Water and power inlet_v8 (Autodesk Fusion 360 design; units mm, degrees)
Autodesk Fusion 360 part; units mm, degrees
sketch "Sketch1" plane through (0, 0, 0) normal (0, 1, 0) x (1, 0, 0)
  line L0 (-30, -30) -> (30, -30)
  line L1 (30, -30) -> (30, 30)
  line L2 (30, 30) -> (-30, 30)
  line L3 (-30, 30) -> (-30, -30)
  line L4 (-30, -30) -> (30, 30) construction
  line L5 (30, -30) -> (-30, 30) construction
  circle A0 centre (10, 0) radius 13.5
  line L6 (10, 0) -> (10, -22.5) construction
  line L7 (10, 0) -> (10, 22.5) construction
  circle A1 centre (10, -22.5) radius 2.25
  circle A2 centre (10, 22.5) radius 2.25
  circle A3 centre (10, 0) radius 17.5
  line L8 (30, -30) -> (24, -30)
  line L9 (24, -30) -> (24, 30)
  line L10 (24, 30) -> (30, 30)
  line L11 (30, 30) -> (30, -30)
  line L12 (-30, -30) -> (-24, -30)
  line L13 (-24, -30) -> (-24, 30)
  line L14 (-24, 30) -> (-30, 30)
  line L15 (-30, 30) -> (-30, -30)
  circle A4 centre (-19, 13) radius 5.6
  line L16 (-11.5, 17.3301) -> (-19, 21.6603)
  line L17 (-19, 21.6603) -> (-26.5, 17.3301)
  line L18 (-26.5, 17.3301) -> (-26.5, 8.6699)
  line L19 (-26.5, 8.6699) -> (-19, 4.3397)
  line L20 (-19, 4.3397) -> (-11.5, 8.6699)
  line L21 (-11.5, 8.6699) -> (-11.5, 17.3301)
  circle A5 centre (10, -22.5) radius 3.75
  circle A6 centre (10, 22.5) radius 3.75
  circle A7 centre (-19, 4.3397) radius 5
  line L22 (-16, 19) -> (-22, 19)
  line L23 (-22, 19) -> (-22, 29)
  line L24 (-22, 29) -> (-16, 29)
  line L25 (-16, 29) -> (-16, 19)
  circle A8 centre (-19, -12) radius 6.25
  line L26 (-28, -27) -> (-10, -27) construction
  line L27 (-10, -27) -> (-10, 3) construction
  line L28 (-10, 3) -> (-28, 3) construction
  line L29 (-28, 3) -> (-28, -27) construction
  line L30 (-28, -27) -> (-10, 3) construction
  line L31 (-10, -27) -> (-28, 3) construction
  circle A9 centre (-10.0486, 22.5) radius 2.55
  circle A10 centre (-10.0486, 22.5) radius 3
  circle A11 centre (-19, -12) radius 10
  line L32 (-22.3912, -17.25) -> (-15.6088, -17.25) construction
  line L33 (-19, -12) -> (-19, -17.25) construction
  line L34 (-19, -17.25) -> (-19.45, -17.25) construction
  line L35 (-19, -17.25) -> (-18.55, -17.25) construction
  line L36 (-18.55, -17.25) -> (-19.45, -17.25)
  line L37 (-19.45, -17.25) -> (-19.45, -18.35)
  line L38 (-19.45, -18.35) -> (-18.55, -18.35)
  line L39 (-18.55, -18.35) -> (-18.55, -17.25)
  point P0 (-19, 13)
  point P1 (-19, -12)
  dimension "d1" = 60
  dimension "d2" = 60
  dimension "d3" = 27
  dimension "d4" = 22.5
  dimension "d5" = 22.5
  dimension "d6" = 4.5
  dimension "d7" = 4.5
  dimension "d18" = 35
  dimension "d19" = 6
  dimension "d20" = 6
  dimension "d24" = 11.2
  dimension "d34" = 7.5
  dimension "d35" = 7.5
  dimension "d36" = 7.5
  dimension "d73" = 10
  dimension "d74" = 12.5
  dimension "d75" = 18
  dimension "d76" = 30
  dimension "d77" = 6
  dimension "d78" = 5.1
  dimension "d85" = 6
  dimension "d91" = 20
  dimension "d92" = 5.25
  dimension "d93" = 0.45
  dimension "d94" = 0.45
  dimension "d95" = 1.1
  constraint horizontal L0
  constraint perpendicular L0 L1
  constraint parallel L0 L2
  constraint parallel L1 L3
  constraint coincident L4 origin
  constraint coincident L5 origin
  constraint coincident A0.centre L6.start
  constraint vertical L6
  constraint parallel L6 L7
  constraint coincident L6.end A1.centre
  constraint coincident L7.end A2.centre
  constraint concentric A0 A3
  constraint horizontal L8
  constraint vertical L9
  constraint horizontal L10
  constraint vertical L11
  constraint horizontal L12
  constraint vertical L13
  constraint horizontal L14
  constraint vertical L15
  constraint coincident P0 A4.centre
  constraint concentric A2 A6
  constraint coincident L19.end L20.start
  constraint tangent L13 A7
  constraint horizontal L22
  constraint vertical L23
  constraint horizontal L24
  constraint vertical L25
  constraint horizontal L26
  constraint perpendicular L26 L27
  constraint parallel L26 L28
  constraint parallel L27 L29
  constraint coincident L30 P1
  constraint coincident L31 P1
  constraint coincident P1 A8.centre
  constraint concentric A9 A10
  constraint concentric A8 A11
  constraint coincident A8 L32.start
  constraint coincident A8 L32.end
  constraint horizontal L32
  constraint midpoint L32 L33.end
  constraint perpendicular L33 L34
  constraint perpendicular L33 L35
  constraint horizontal L36
  constraint vertical L37
  constraint horizontal L38
  constraint vertical L39
  measures "d1" distance of L1.end L2.end
  measures "d2" distance of L0.end L1.end L2.end
  measures "d3" diameter of A0
  measures "d4" distance of A0.centre L6.end
  measures "d5" distance of A0.centre L7.end
  measures "d6" diameter of A1
  measures "d7" diameter of A2
  measures "d18" diameter of A3
  measures "d19" distance of L0.end L8.end
  measures "d20" distance of L0.start L12.end L2.end
  measures "d24" diameter of A4
  measures "d34" distance of P0 L21
  measures "d35" diameter of A5
  measures "d36" diameter of A6
  measures "d73" distance of L22.start L24.end
  measures "d74" diameter of A8
  measures "d75" distance of L27.end L28.end
  measures "d76" distance of L26.end L27.end
  measures "d77" distance of P0 L22
  measures "d78" diameter of A9
  measures "d85" diameter of A10
  measures "d91" diameter of A11
  measures "d92" distance of P1 L32
  measures "d93" distance of L33.end L34.end
  measures "d94" distance of L33.end L35.end
  measures "d95" distance of L35.end L38.end
extrude "Extrude1" add sketch "Sketch1" along normal blind 14 contours L0 L2 L3 L12 L13 L14 L15 L17 L18 L19 A11 | L0 L2 A3 L9 L13 L16 L17 L20 L21 A7 L23 L24 L25 A11 | L0 L1 L2 A3 L8 L9 L10 L11 | L13 A8 A11 | L13 A8 A11 L37 L38 L39 | A3 L9 | A3 L9 | L13 A8 | L13 A8 L36 L37 L39 | A8 L36 L37 L39 | A8 L37 L38 L39 | L13 L19 A7 | A5 | A6 | A9 | A10
sketch "Sketch2" plane through (0, 0, 30) normal (0, 0, 1) x (-1, 0, 0)
  line L0 (-30, 0) -> (-30, -14)
  line L1 (-30, -14) -> (30, -14)
  line L2 (30, -14) -> (30, 0)
  line L3 (31.85, 1.95) -> (33.4186, 1.95)
  line L4 (30.114, 0.8971) -> (31.423, -0.4137)
  arc A0 (31.423, -0.4137) -> (31.85, -0.2372) centre (31.6, -0.2372) ccw
  line L5 (31.85, -8.95) -> (31.85, -6.7628)
  line L6 (33.4186, -8.95) -> (31.85, -8.95)
  line L7 (36.05, -6.3186) -> (33.4186, -8.95)
  line L8 (31.85, -0.2372) -> (31.85, 1.95)
  arc A1 (31.85, -6.7628) -> (31.4232, -6.5861) centre (31.6, -6.7628) ccw
  line L9 (31.4232, -6.5861) -> (30.1424, -7.8668)
  line L10 (33.4186, 1.95) -> (36.05, -0.6814)
  line L11 (36.05, -0.6814) -> (36.05, -6.3186)
  line L12 (30.1571, -7.8522) -> (30, -7.8522)
  line L13 (30, -7.8522) -> (30, 0.8812)
  line L14 (30, 0.8812) -> (30.1299, 0.8812)
  line L15 (40, -9) -> (-35, -9) construction
  line L16 (0, -16) -> (0, 2) construction
  line L17 (-30.114, 0.8971) -> (-31.423, -0.4137)
  line L18 (-31.85, -0.2372) -> (-31.85, 1.95)
  line L19 (-31.4232, -6.5861) -> (-30.1424, -7.8668)
  line L20 (-30, 0.8812) -> (-30.1299, 0.8812)
  line L21 (-30.1571, -7.8522) -> (-30, -7.8522)
  line L22 (-33.4186, 1.95) -> (-36.05, -0.6814)
  line L23 (-31.85, 1.95) -> (-33.4186, 1.95)
  line L24 (-33.4186, -8.95) -> (-31.85, -8.95)
  line L25 (-31.85, -8.95) -> (-31.85, -6.7628)
  arc A2 (-31.85, -0.2372) -> (-31.423, -0.4137) centre (-31.6, -0.2372) ccw
  line L26 (-30, -7.8522) -> (-30, 0.8812)
  line L27 (-36.05, -6.3186) -> (-33.4186, -8.95)
  line L28 (-36.05, -0.6814) -> (-36.05, -6.3186)
  arc A3 (-31.4232, -6.5861) -> (-31.85, -6.7628) centre (-31.6, -6.7628) ccw
  point P0 (30, -3.5)
  point P1 (-30, 0)
  point P2 (-30, -3.5)
  constraint coincident L9 L12.start
  constraint coincident L4 L14.end
  constraint tangent A0 L8
  constraint tangent L5 A1
  constraint tangent A1 L9
  constraint horizontal L15
  constraint perpendicular L1 L16
  constraint symmetric L2.end L16 L0.start
  constraint symmetric L7.start L16 L27.start
  constraint symmetric L3.end L16 L22.start
  constraint symmetric A1.end L16 L19.start
  constraint symmetric P0 L16 P2
  constraint symmetric L4.start L16 L17.start
  constraint symmetric L4.end L16 L17.end
  constraint symmetric L9.end L16 L19.end
  constraint symmetric L10.end L16 L22.end
  constraint symmetric L3.start L16 L18.end
  constraint symmetric A0.end L16 L18.start
  constraint symmetric L6.start L16 L24.start
  constraint symmetric L5.start L16 L24.end
  constraint symmetric L5.end L16 L25.end
  constraint symmetric A0 L16 A2
  constraint symmetric A1 L16 A3
  constraint symmetric L12.start L16 L21.start
  constraint symmetric L12.end L16 L21.end
  constraint symmetric L13.end L16 L20.start
  constraint symmetric L14.end L16 L20.end
extrude "Extrude2" add sketch "Sketch2" against normal blind 60
extrude "Extrude3" add sketch "Sketch1" against normal blind 7 contours L0 L2 L3 L12 L13 L14 L15 L17 L18 L19 A11 | L0 L1 L2 A3 L8 L9 L10 L11 | L13 A8 A11 | L13 A8
extrude "Extrude4" add sketch "Sketch1" along normal blind 9 from surface at 5 contours L13 A4 L16 L17 L20 L21 A7 L22 L23 L25 | L13 A4 L17 L18 L19 | L19 L20 A7 | L16 L17 L23 L24 L25 | L16 L17 L22 L23 L25 | L13 A4 L19 A7 | A4 L19 L20 A7
fillet "Fillet3" radius 6 5 edges at (-24, -7, 11.3868) (-24, -7, -24.3868) (24, -7, 20.25) (-24, -7, -24.3868) (24, -7, -20.25)
extrude "Extrude5" cut sketch "Sketch1" along normal blind 4 contours A5 | A6
fillet "Fillet4" radius 5 2 edges at (-23.3301, 2.5, -6.8397) (-14.6699, 2.5, -6.8397)
sketch "Sketch3" plane through (0, 14, 0) normal (0, 1, 0) x (-1, 0, 0)
  circle A0 centre (19, -13) radius 5.6
  circle A1 centre (-10, 22.5) radius 2.25
  circle A2 centre (-10, 0) radius 13.5
  circle A3 centre (-10, -22.5) radius 2.25
  line L0 (-30, -30) -> (30, -30)
  line L1 (30, -30) -> (30, 30)
  line L2 (30, 30) -> (-30, 30)
  line L3 (-30, 30) -> (-30, -30)
  circle A4 centre (19, -13) radius 8
  dimension "d41" = 16
  constraint concentric A0 A4
  measures "d41" diameter of A4
extrude "Extrude6" cut sketch "Sketch3" against normal blind 4.8 contours A4
extrude "Extrude7" add sketch "Sketch3" along normal blind 0.2 from surface at -5 contours A0 | A4
sketch "Sketch4" plane through (0, 0, 30) normal (0, 0, 1) x (-1, 0, 0)
  arc A0 (-24, 1) -> (-30, 7) centre (-30, 1) ccw
  line L0 (-30, 7) -> (-30, 0.8812)
  line L1 (-30, 0.8812) -> (-30.1299, 0.8812)
  line L2 (-30.1299, 0.8812) -> (-31.423, -0.4137)
  arc A1 (-31.85, -0.2372) -> (-31.423, -0.4137) centre (-31.6, -0.2372) ccw
  line L3 (-31.85, -0.2372) -> (-31.85, 1.95)
  line L4 (-31.85, 1.95) -> (-33.4186, 1.95)
  line L5 (-33.4186, 1.95) -> (-36.05, -0.6814)
  line L6 (-36.05, -0.6814) -> (-36.05, -6.3186)
  line L7 (-36.05, -6.3186) -> (-33.4186, -8.95)
  line L8 (-33.4186, -8.95) -> (-31.85, -8.95)
  line L9 (-31.85, -8.95) -> (-31.85, -6.7628)
  arc A2 (-31.4232, -6.5861) -> (-31.85, -6.7628) centre (-31.6, -6.7628) ccw
  line L10 (-31.4232, -6.5861) -> (-30.1571, -7.8522)
  line L11 (-30.1571, -7.8522) -> (-30, -7.8522)
  line L12 (-30, -7.8522) -> (-30, -14)
  line L13 (-30, -14) -> (30, -14)
  line L14 (30, -14) -> (30, -7.8522)
  line L15 (30, -7.8522) -> (30.1571, -7.8522)
  line L16 (30.1571, -7.8522) -> (31.4232, -6.5861)
  arc A3 (31.85, -6.7628) -> (31.4232, -6.5861) centre (31.6, -6.7628) ccw
  line L17 (31.85, -6.7628) -> (31.85, -8.95)
  line L18 (31.85, -8.95) -> (33.4186, -8.95)
  line L19 (33.4186, -8.95) -> (36.05, -6.3186)
  line L20 (36.05, -6.3186) -> (36.05, -0.6814)
  line L21 (36.05, -0.6814) -> (33.4186, 1.95)
  line L22 (33.4186, 1.95) -> (31.85, 1.95)
  line L23 (31.85, 1.95) -> (31.85, -0.2372)
  arc A4 (31.423, -0.4137) -> (31.85, -0.2372) centre (31.6, -0.2372) ccw
  line L24 (31.423, -0.4137) -> (30.1299, 0.8812)
  line L25 (30.1299, 0.8812) -> (30, 0.8812)
  line L26 (30, 0.8812) -> (30, 7)
  arc A5 (30, 7) -> (24, 1) centre (30, 1) ccw
  line L27 (24, 1) -> (24, 0)
  line L28 (24, 0) -> (-24, 0)
  line L29 (-24, 0) -> (-24, 1)
  line L30 (36.05, -3.5) -> (-36.05, -3.5) construction
  line L31 (-22.8393, -7.4) -> (-17.1607, -7.4)
  line L32 (3.2628, 4.7) -> (5.5, 4.7)
  line L33 (17.1607, -7.4) -> (22.8393, -7.4)
  line L34 (-14.5, 3.0607) -> (-17.1607, 0.4)
  line L35 (-7.3, 4.7) -> (-7.3, 2.7393)
  line L36 (-4.9, 6.5) -> (-15.1, 6.5)
  arc A6 (4.9, 6.5) -> (4.4022, 6.3222) centre (4.8416, 5.8778) ccw
  line L37 (-7.3, 2.7393) -> (-3.9, -0.6607)
  line L38 (15.1, 6.5) -> (4.9, 6.5)
  line L39 (-16.1, -0.6607) -> (-12.7, 2.7393)
  line L40 (5.5, 4.7) -> (5.5, 3.0607)
  line L41 (-16.1, -0.6607) -> (-12.7, 2.7393)
  line L42 (-12.7, 2.7393) -> (-12.7, 4.7)
  line L43 (-3.1214, 5.0414) -> (-4.4022, 6.3222)
  line L44 (-5.5, 3.0607) -> (-5.5, 4.7)
  arc A7 (16.7372, 4.7) -> (16.8786, 5.0414) centre (16.7372, 4.9) ccw
  line L45 (-5.5, 4.7) -> (-3.2628, 4.7)
  line L46 (14.5, 4.7) -> (16.7372, 4.7)
  line L47 (17.1607, -7.4) -> (22.8393, -7.4)
  arc A8 (-4.9, -13.5) -> (-4.4022, -13.3222) centre (-4.8409, -12.8798) ccw
  line L48 (-16.8786, -12.0414) -> (-15.5978, -13.3222)
  line L49 (-16.1, -6.3393) -> (-16.1, -0.6607)
  line L50 (-17.1607, -7.4) -> (-14.5, -10.0607)
  line L51 (-14.5, -11.7) -> (-16.7372, -11.7)
  line L52 (-7.3, -9.7393) -> (-7.3, -11.7)
  line L53 (-12.7, -9.7393) -> (-16.1, -6.3393)
  line L54 (-7.3, -9.7393) -> (-7.3, -11.7)
  arc A9 (-16.7372, -11.7) -> (-16.8786, -12.0414) centre (-16.7372, -11.9) ccw
  line L55 (-14.5, -10.0607) -> (-14.5, -11.7)
  line L56 (-14.5, -11.7) -> (-16.7372, -11.7)
  line L57 (-12.7, -11.7) -> (-12.7, -9.7393)
  line L58 (-12.7, -9.7393) -> (-16.1, -6.3393)
  line L59 (-22.8393, 0.4) -> (-25.5, 3.0607)
  line L60 (12.7, 2.7393) -> (16.1, -0.6607)
  line L61 (16.1, -0.6607) -> (16.1, -6.3393)
  line L62 (29.8222, -7.9022) -> (28.5414, -6.6214)
  line L63 (-28.2, 2) -> (-26.5607, 2)
  line L64 (23.9, -6.3393) -> (23.9, -0.6607)
  arc A10 (28.2, -0.2372) -> (28.5414, -0.3786) centre (28.4, -0.2372) ccw
  line L65 (12.7, 2.7393) -> (16.1, -0.6607)
  line L66 (22.8393, 0.4) -> (17.1607, 0.4)
  line L67 (5.5, 3.0607) -> (2.8393, 0.4)
  arc A11 (23.2628, -11.7) -> (23.1214, -12.0414) centre (23.2628, -11.9) ccw
  line L68 (25.5, 3.0607) -> (22.8393, 0.4)
  line L69 (15.1, 6.5) -> (4.9, 6.5)
  arc A12 (3.1214, 5.0414) -> (3.2628, 4.7) centre (3.2628, 4.9) ccw
  line L70 (4.4022, 6.3222) -> (3.1214, 5.0414)
  circle A13 centre (20, -3.5) radius 2.1
  line L71 (23.9, -6.3393) -> (23.9, -0.6607)
  line L72 (5.5, 4.7) -> (5.5, 3.0607)
  line L73 (3.9, -6.3393) -> (3.9, -0.6607)
  line L74 (-17.1607, 0.4) -> (-22.8393, 0.4)
  line L75 (14.5, 3.0607) -> (14.5, 4.7)
  line L76 (-23.9, -0.6607) -> (-23.9, -6.3393)
  line L77 (-22.8393, -7.4) -> (-17.1607, -7.4)
  line L78 (16.1, -0.6607) -> (16.1, -6.3393)
  line L79 (-25.5, -11.7) -> (-25.5, -10.0607)
  arc A14 (15.5978, 6.3222) -> (15.1, 6.5) centre (15.1584, 5.8778) ccw
  line L80 (7.3, 2.7393) -> (7.3, 4.7)
  arc A15 (30, 6) -> (29.5, 6.5) centre (29.5, 6) ccw
  line L81 (16.8786, 5.0414) -> (15.5978, 6.3222)
  arc A16 (-23.2628, 4.7) -> (-23.1214, 5.0414) centre (-23.2628, 4.9) ccw
  arc A17 (29.8222, 0.9022) -> (30, 1.3314) centre (29.3929, 1.3314) ccw
  line L82 (-23.9, -0.6607) -> (-23.9, -6.3393)
  arc A18 (4.9, 6.5) -> (4.4022, 6.3222) centre (4.8416, 5.8778) ccw
  line L83 (12.7, 4.7) -> (12.7, 2.7393)
  line L84 (-7.3, 2.7393) -> (-3.9, -0.6607)
  circle A19 centre (-20, -3.5) radius 2.1
  line L85 (-17.1607, 0.4) -> (-22.8393, 0.4)
  line L86 (26.5607, 2) -> (28.2, 2)
  line L87 (22.8393, -7.4) -> (25.5, -10.0607)
  line L88 (24.8314, -13.5) -> (29.5, -13.5)
  line L89 (26.5607, -9) -> (23.9, -6.3393)
  line L90 (22.8393, 0.4) -> (17.1607, 0.4)
  arc A20 (16.7372, 4.7) -> (16.8786, 5.0414) centre (16.7372, 4.9) ccw
  line L91 (3.9, -6.3393) -> (3.9, -0.6607)
  line L92 (-25.5, 3.0607) -> (-25.5, 4.7)
  line L93 (4.4022, 6.3222) -> (3.1214, 5.0414)
  arc A21 (24.9, 6.5) -> (24.4022, 6.3222) centre (24.8416, 5.8778) ccw
  line L94 (5.5, 3.0607) -> (2.8393, 0.4)
  line L95 (-30, 6) -> (-30, 1.3314)
  arc A22 (28.5414, -6.6214) -> (28.2, -6.7628) centre (28.4, -6.7628) ccw
  line L96 (24.8314, -13.5) -> (29.5, -13.5)
  arc A23 (28.2, -0.2372) -> (28.5414, -0.3786) centre (28.4, -0.2372) ccw
  arc A24 (-30, 1.3314) -> (-29.8222, 0.9022) centre (-29.3929, 1.3314) ccw
  line L97 (12.7, 4.7) -> (12.7, 2.7393)
  line L98 (25.5, -10.0607) -> (25.5, -11.7)
  line L99 (3.9, -0.6607) -> (7.3, 2.7393)
  line L100 (28.2, 2) -> (28.2, -0.2372)
  line L101 (-24.4022, -13.3222) -> (-23.1214, -12.0414)
  line L102 (3.2628, 4.7) -> (5.5, 4.7)
  line L103 (28.5414, -0.3786) -> (29.8222, 0.9022)
  arc A25 (-23.1214, -12.0414) -> (-23.2628, -11.7) centre (-23.2628, -11.9) ccw
  line L104 (16.1, -6.3393) -> (12.7, -9.7393)
  line L105 (25.5, 3.0607) -> (22.8393, 0.4)
  arc A26 (-24.4022, 6.3222) -> (-24.9, 6.5) centre (-24.8416, 5.8778) ccw
  arc A27 (3.1214, 5.0414) -> (3.2628, 4.7) centre (3.2628, 4.9) ccw
  line L106 (7.3, 4.7) -> (12.7, 4.7)
  arc A28 (23.1214, 5.0414) -> (23.2628, 4.7) centre (23.2628, 4.9) ccw
  arc A29 (-30, 1.3314) -> (-29.8222, 0.9022) centre (-29.3929, 1.3314) ccw
  line L107 (-25.5, 4.7) -> (-23.2628, 4.7)
  line L108 (14.5, 3.0607) -> (14.5, 4.7)
  line L109 (-28.2, -0.2372) -> (-28.2, 2)
  line L110 (26.5607, -9) -> (23.9, -6.3393)
  line L111 (30, -13) -> (30, -8.3314)
  line L112 (23.2628, 4.7) -> (25.5, 4.7)
  line L113 (3.9, -0.6607) -> (7.3, 2.7393)
  arc A30 (29.5, -13.5) -> (30, -13) centre (29.5, -13) ccw
  arc A31 (24.9, 6.5) -> (24.4022, 6.3222) centre (24.8416, 5.8778) ccw
  arc A32 (29.5, -13.5) -> (30, -13) centre (29.5, -13) ccw
  arc A33 (-29.5, 6.5) -> (-30, 6) centre (-29.5, 6) ccw
  arc A34 (23.1214, 5.0414) -> (23.2628, 4.7) centre (23.2628, 4.9) ccw
  arc A35 (16.8786, -12.0414) -> (16.7372, -11.7) centre (16.7372, -11.9) ccw
  line L114 (30, -13) -> (30, -8.3314)
  line L115 (7.3, 2.7393) -> (7.3, 4.7)
  line L116 (23.2628, 4.7) -> (25.5, 4.7)
  arc A36 (-24.4022, 6.3222) -> (-24.9, 6.5) centre (-24.8416, 5.8778) ccw
  line L117 (23.1214, -12.0414) -> (24.4022, -13.3222)
  line L118 (-25.5, 3.0607) -> (-25.5, 4.7)
  arc A37 (-24.8314, -13.5) -> (-24.4022, -13.3222) centre (-24.8314, -12.8929) ccw
  line L119 (29.8222, -7.9022) -> (28.5414, -6.6214)
  arc A38 (-28.2, -6.7628) -> (-28.5414, -6.6214) centre (-28.4, -6.7628) ccw
  arc A39 (-29.5, 6.5) -> (-30, 6) centre (-29.5, 6) ccw
  line L120 (16.8786, 5.0414) -> (15.5978, 6.3222)
  arc A40 (28.5414, -6.6214) -> (28.2, -6.7628) centre (28.4, -6.7628) ccw
  line L121 (25.5, -10.0607) -> (25.5, -11.7)
  line L122 (-26.5607, 2) -> (-23.9, -0.6607)
  line L123 (7.3, 4.7) -> (12.7, 4.7)
  line L124 (28.2, -9) -> (26.5607, -9)
  arc A41 (15.5978, 6.3222) -> (15.1, 6.5) centre (15.1584, 5.8778) ccw
  arc A42 (-30, -13) -> (-29.5, -13.5) centre (-29.5, -13) ccw
  line L125 (-25.5, 4.7) -> (-23.2628, 4.7)
  arc A43 (-24.8314, -13.5) -> (-24.4022, -13.3222) centre (-24.8314, -12.8929) ccw
  line L126 (17.1607, 0.4) -> (14.5, 3.0607)
  line L127 (25.5, 4.7) -> (25.5, 3.0607)
  line L128 (28.5414, -0.3786) -> (29.8222, 0.9022)
  line L129 (-24.9, 6.5) -> (-29.5, 6.5)
  arc A44 (24.4022, -13.3222) -> (24.8314, -13.5) centre (24.8314, -12.8929) ccw
  arc A45 (23.2628, -11.7) -> (23.1214, -12.0414) centre (23.2628, -11.9) ccw
  arc A46 (30, 6) -> (29.5, 6.5) centre (29.5, 6) ccw
  arc A47 (24.4022, -13.3222) -> (24.8314, -13.5) centre (24.8314, -12.8929) ccw
  line L130 (-28.5414, -6.6214) -> (-29.8222, -7.9022)
  line L131 (-28.2, 2) -> (-26.5607, 2)
  line L132 (-29.8222, 0.9022) -> (-28.5414, -0.3786)
  line L133 (16.1, -6.3393) -> (12.7, -9.7393)
  line L134 (-25.5, -11.7) -> (-25.5, -10.0607)
  arc A48 (-30, -13) -> (-29.5, -13.5) centre (-29.5, -13) ccw
  line L135 (28.2, 2) -> (28.2, -0.2372)
  line L136 (7.3, -9.7393) -> (3.9, -6.3393)
  line L137 (-29.5, -13.5) -> (-24.8314, -13.5)
  line L138 (24.4022, 6.3222) -> (23.1214, 5.0414)
  arc A49 (30, -8.3314) -> (29.8222, -7.9022) centre (29.3929, -8.3314) ccw
  line L139 (23.1214, -12.0414) -> (24.4022, -13.3222)
  line L140 (-22.8393, 0.4) -> (-25.5, 3.0607)
  line L141 (-24.4022, -13.3222) -> (-23.1214, -12.0414)
  line L142 (25.5, -11.7) -> (23.2628, -11.7)
  line L143 (25.5, -11.7) -> (23.2628, -11.7)
  arc A50 (-28.5414, -0.3786) -> (-28.2, -0.2372) centre (-28.4, -0.2372) ccw
  line L144 (12.7, -9.7393) -> (12.7, -11.7)
  line L145 (-28.5414, -6.6214) -> (-29.8222, -7.9022)
  line L146 (-26.5607, -9) -> (-28.2, -9)
  line L147 (25.5, 4.7) -> (25.5, 3.0607)
  line L148 (-23.2628, -11.7) -> (-25.5, -11.7)
  line L149 (-24.9, 6.5) -> (-29.5, 6.5)
  line L150 (14.5, 4.7) -> (16.7372, 4.7)
  arc A51 (-28.5414, -0.3786) -> (-28.2, -0.2372) centre (-28.4, -0.2372) ccw
  line L151 (-23.1214, 5.0414) -> (-24.4022, 6.3222)
  line L152 (22.8393, -7.4) -> (25.5, -10.0607)
  arc A52 (29.8222, 0.9022) -> (30, 1.3314) centre (29.3929, 1.3314) ccw
  line L153 (-28.2, -0.2372) -> (-28.2, 2)
  arc A53 (-29.8222, -7.9022) -> (-30, -8.3314) centre (-29.3929, -8.3314) ccw
  line L154 (16.7372, -11.7) -> (14.5, -11.7)
  arc A54 (-23.2628, 4.7) -> (-23.1214, 5.0414) centre (-23.2628, 4.9) ccw
  line L155 (-25.5, -10.0607) -> (-22.8393, -7.4)
  line L156 (23.9, -0.6607) -> (26.5607, 2)
  line L157 (7.3, -11.7) -> (7.3, -9.7393)
  line L158 (5.5, -10.0607) -> (5.5, -11.7)
  line L159 (23.9, -0.6607) -> (26.5607, 2)
  line L160 (2.8393, -7.4) -> (5.5, -10.0607)
  line L161 (14.5, -10.0607) -> (17.1607, -7.4)
  line L162 (29.5, 6.5) -> (24.9, 6.5)
  line L163 (-23.1214, 5.0414) -> (-24.4022, 6.3222)
  line L164 (26.5607, 2) -> (28.2, 2)
  arc A55 (30, -8.3314) -> (29.8222, -7.9022) centre (29.3929, -8.3314) ccw
  line L165 (30, 1.3314) -> (30, 6)
  line L166 (14.5, -11.7) -> (14.5, -10.0607)
  line L167 (28.2, -9) -> (26.5607, -9)
  line L168 (28.2, -6.7628) -> (28.2, -9)
  line L169 (28.2, -6.7628) -> (28.2, -9)
  line L170 (-23.9, -6.3393) -> (-26.5607, -9)
  line L171 (17.1607, 0.4) -> (14.5, 3.0607)
  line L172 (-29.8222, 0.9022) -> (-28.5414, -0.3786)
  line L173 (4.9, -13.5) -> (15.1, -13.5)
  line L174 (14.5, -11.7) -> (14.5, -10.0607)
  arc A56 (3.2628, -11.7) -> (3.1214, -12.0414) centre (3.2628, -11.9) ccw
  line L175 (24.4022, 6.3222) -> (23.1214, 5.0414)
  line L176 (-30, 6) -> (-30, 1.3314)
  arc A57 (-28.2, -6.7628) -> (-28.5414, -6.6214) centre (-28.4, -6.7628) ccw
  arc A58 (16.8786, -12.0414) -> (16.7372, -11.7) centre (16.7372, -11.9) ccw
  line L177 (-23.2628, -11.7) -> (-25.5, -11.7)
  line L178 (-29.5, -13.5) -> (-24.8314, -13.5)
  line L179 (5.5, -11.7) -> (3.2628, -11.7)
  line L180 (15.5978, -13.3222) -> (16.8786, -12.0414)
  arc A59 (4.4022, -13.3222) -> (4.9, -13.5) centre (4.8416, -12.8778) ccw
  line L181 (3.1214, -12.0414) -> (4.4022, -13.3222)
  arc A60 (4.4022, -13.3222) -> (4.9, -13.5) centre (4.8416, -12.8778) ccw
  line L182 (7.3, -11.7) -> (7.3, -9.7393)
  line L183 (29.5, 6.5) -> (24.9, 6.5)
  line L184 (-26.5607, 2) -> (-23.9, -0.6607)
  line L185 (-28.2, -9) -> (-28.2, -6.7628)
  line L186 (16.7372, -11.7) -> (14.5, -11.7)
  arc A61 (3.2628, -11.7) -> (3.1214, -12.0414) centre (3.2628, -11.9) ccw
  line L187 (30, 1.3314) -> (30, 6)
  line L188 (-28.2, -9) -> (-28.2, -6.7628)
  line L189 (-25.5, -10.0607) -> (-22.8393, -7.4)
  line L190 (-23.9, -6.3393) -> (-26.5607, -9)
  line L191 (3.1214, -12.0414) -> (4.4022, -13.3222)
  arc A62 (-23.1214, -12.0414) -> (-23.2628, -11.7) centre (-23.2628, -11.9) ccw
  line L192 (12.7, -11.7) -> (7.3, -11.7)
  line L193 (2.8393, -7.4) -> (5.5, -10.0607)
  line L194 (12.7, -11.7) -> (7.3, -11.7)
  line L195 (12.7, -9.7393) -> (12.7, -11.7)
  line L196 (-26.5607, -9) -> (-28.2, -9)
  line L197 (4.9, -13.5) -> (15.1, -13.5)
  line L198 (5.5, -10.0607) -> (5.5, -11.7)
  line L199 (-30, -8.3314) -> (-30, -13)
  line L200 (7.3, -9.7393) -> (3.9, -6.3393)
  line L201 (14.5, -10.0607) -> (17.1607, -7.4)
  line L202 (-30, -8.3314) -> (-30, -13)
  arc A63 (15.1, -13.5) -> (15.5978, -13.3222) centre (15.1584, -12.8778) ccw
  line L203 (15.5978, -13.3222) -> (16.8786, -12.0414)
  arc A64 (-29.8222, -7.9022) -> (-30, -8.3314) centre (-29.3929, -8.3314) ccw
  line L204 (5.5, -11.7) -> (3.2628, -11.7)
  arc A65 (15.1, -13.5) -> (15.5978, -13.3222) centre (15.1584, -12.8778) ccw
  line L205 (-14.5, 4.7) -> (-14.5, 3.0607)
  line L206 (-4.9, 6.5) -> (-15.1, 6.5)
  line L207 (-3.1214, 5.0414) -> (-4.4022, 6.3222)
  line L208 (-7.3, 4.7) -> (-7.3, 2.7393)
  line L209 (-5.5, 3.0607) -> (-5.5, 4.7)
  line L210 (-12.7, 2.7393) -> (-12.7, 4.7)
  line L211 (-2.8393, 0.4) -> (-5.5, 3.0607)
  line L212 (-5.5, 4.7) -> (-3.2628, 4.7)
  line L213 (-15.5978, 6.3222) -> (-16.8786, 5.0414)
  arc A66 (-16.8786, 5.0414) -> (-16.7372, 4.7) centre (-16.7372, 4.9) ccw
  line L214 (-16.7372, 4.7) -> (-14.5, 4.7)
  line L215 (-2.8393, 0.4) -> (-5.5, 3.0607)
  line L216 (-14.5, 3.0607) -> (-17.1607, 0.4)
  arc A67 (-4.9, -13.5) -> (-4.4022, -13.3222) centre (-4.8409, -12.8798) ccw
  arc A68 (-3.1214, -12.0414) -> (-3.2628, -11.7) centre (-3.2628, -11.9) ccw
  line L217 (-2.8393, -7.4) -> (2.8393, -7.4)
  line L218 (-3.9, -0.6607) -> (-3.9, -6.3393)
  line L219 (-4.4022, -13.3222) -> (-3.1214, -12.0414)
  line L220 (-4.4022, -13.3222) -> (-3.1214, -12.0414)
  line L221 (-3.9, -6.3393) -> (-7.3, -9.7393)
  circle A69 centre (0, -3.5) radius 2.1
  line L222 (-15.1, -13.5) -> (-4.9, -13.5)
  line L223 (-15.1, -13.5) -> (-4.9, -13.5)
  line L224 (-2.8393, -7.4) -> (2.8393, -7.4)
  line L225 (-3.9, -6.3393) -> (-7.3, -9.7393)
  line L226 (2.8393, 0.4) -> (-2.8393, 0.4)
  line L227 (2.8393, 0.4) -> (-2.8393, 0.4)
  arc A70 (-15.5978, -13.3222) -> (-15.1, -13.5) centre (-15.1591, -12.8798) ccw
  line L228 (-16.8786, -12.0414) -> (-15.5978, -13.3222)
  line L229 (-14.5, -10.0607) -> (-14.5, -11.7)
  line L230 (-7.3, -11.7) -> (-12.7, -11.7)
  line L231 (-12.7, -11.7) -> (-12.7, -9.7393)
  line L232 (-3.9, -0.6607) -> (-3.9, -6.3393)
  line L233 (-5.5, -10.0607) -> (-2.8393, -7.4)
  line L234 (-3.2628, -11.7) -> (-5.5, -11.7)
  line L235 (-5.5, -11.7) -> (-5.5, -10.0607)
  line L236 (-5.5, -10.0607) -> (-2.8393, -7.4)
  line L237 (-16.1, -6.3393) -> (-16.1, -0.6607)
  arc A71 (-16.7372, -11.7) -> (-16.8786, -12.0414) centre (-16.7372, -11.9) ccw
  line L238 (-17.1607, -7.4) -> (-14.5, -10.0607)
  arc A72 (-15.5978, -13.3222) -> (-15.1, -13.5) centre (-15.1591, -12.8798) ccw
  line L239 (-7.3, -11.7) -> (-12.7, -11.7)
  line L240 (-12.7, 4.7) -> (-7.3, 4.7)
  arc A73 (-15.1, 6.5) -> (-15.5978, 6.3222) centre (-15.1584, 5.8778) ccw
  line L241 (-16.7372, 4.7) -> (-14.5, 4.7)
  line L242 (-12.7, 4.7) -> (-7.3, 4.7)
  arc A74 (-4.4022, 6.3222) -> (-4.9, 6.5) centre (-4.8416, 5.8778) ccw
  arc A75 (-3.2628, 4.7) -> (-3.1214, 5.0414) centre (-3.2628, 4.9) ccw
  line L243 (-15.5978, 6.3222) -> (-16.8786, 5.0414)
  arc A76 (-16.8786, 5.0414) -> (-16.7372, 4.7) centre (-16.7372, 4.9) ccw
  arc A77 (-15.1, 6.5) -> (-15.5978, 6.3222) centre (-15.1584, 5.8778) ccw
  arc A78 (-4.4022, 6.3222) -> (-4.9, 6.5) centre (-4.8416, 5.8778) ccw
  line L244 (-14.5, 4.7) -> (-14.5, 3.0607)
  arc A79 (-3.2628, 4.7) -> (-3.1214, 5.0414) centre (-3.2628, 4.9) ccw
  line L245 (-5.5, -11.7) -> (-5.5, -10.0607)
  arc A80 (-3.1214, -12.0414) -> (-3.2628, -11.7) centre (-3.2628, -11.9) ccw
  line L246 (-3.2628, -11.7) -> (-5.5, -11.7)
  line L247 (29.5, 6.5) -> (-29.5, 6.5)
  arc A81 (-29.5, 6.6) -> (-30.1, 6) centre (-29.5, 6) ccw
  line L248 (-30.1, 6) -> (-30.1, 1.3314)
  arc A82 (-30.1, 1.3314) -> (-29.8929, 0.8315) centre (-29.3929, 1.3314) ccw
  line L249 (-29.8929, 0.8315) -> (-28.6121, -0.4493)
  arc A83 (-28.6121, -0.4493) -> (-28.1, -0.2372) centre (-28.4, -0.2372) ccw
  line L250 (-28.1, -0.2372) -> (-28.1, 1.9)
  line L251 (-28.1, 1.9) -> (-26.6021, 1.9)
  line L252 (-26.6021, 1.9) -> (-24, -0.7021)
  line L253 (-24, -0.7021) -> (-24, -6.2979)
  line L254 (-24, -6.2979) -> (-26.6021, -8.9)
  line L255 (-26.6021, -8.9) -> (-28.1, -8.9)
  line L256 (-28.1, -8.9) -> (-28.1, -6.7628)
  arc A84 (-28.1, -6.7628) -> (-28.6121, -6.5507) centre (-28.4, -6.7628) ccw
  line L257 (-28.6121, -6.5507) -> (-29.8929, -7.8315)
  arc A85 (-29.8929, -7.8315) -> (-30.1, -8.3314) centre (-29.3929, -8.3314) ccw
  line L258 (-30.1, -8.3314) -> (-30.1, -13)
  arc A86 (-30.1, -13) -> (-29.5, -13.6) centre (-29.5, -13) ccw
  line L259 (-29.5, -13.6) -> (-24.8314, -13.6)
  arc A87 (-24.8314, -13.6) -> (-24.3315, -13.3929) centre (-24.8314, -12.8929) ccw
  line L260 (-24.3315, -13.3929) -> (-23.0507, -12.1121)
  arc A88 (-23.0507, -12.1121) -> (-23.2628, -11.6) centre (-23.2628, -11.9) ccw
  line L261 (-23.2628, -11.6) -> (-25.4, -11.6)
  line L262 (-25.4, -11.6) -> (-25.4, -10.1021)
  line L263 (-25.4, -10.1021) -> (-22.7979, -7.5)
  line L264 (-22.7979, -7.5) -> (-17.2021, -7.5)
  line L265 (-17.2021, -7.5) -> (-14.6, -10.1021)
  line L266 (-14.6, -10.1021) -> (-14.6, -11.6)
  line L267 (-14.6, -11.6) -> (-16.7372, -11.6)
  arc A89 (-16.7372, -11.6) -> (-16.9493, -12.1121) centre (-16.7372, -11.9) ccw
  line L268 (-16.9493, -12.1121) -> (-15.6715, -13.3899)
  arc A90 (-15.6715, -13.3899) -> (-15.0954, -13.6) centre (-15.1591, -12.8798) ccw
  line L269 (-15.0954, -13.6) -> (-4.9046, -13.6)
  arc A91 (-4.9046, -13.6) -> (-4.3308, -13.3922) centre (-4.8409, -12.8798) ccw
  line L270 (-4.3308, -13.3922) -> (-3.0507, -12.1121)
  arc A92 (-3.0507, -12.1121) -> (-3.2628, -11.6) centre (-3.2628, -11.9) ccw
  line L271 (-3.2628, -11.6) -> (-5.4, -11.6)
  line L272 (-5.4, -11.6) -> (-5.4, -10.1021)
  line L273 (-5.4, -10.1021) -> (-2.7979, -7.5)
  line L274 (-2.7979, -7.5) -> (2.7979, -7.5)
  line L275 (2.7979, -7.5) -> (5.4, -10.1021)
  line L276 (5.4, -10.1021) -> (5.4, -11.6)
  line L277 (5.4, -11.6) -> (3.2628, -11.6)
  arc A93 (3.2628, -11.6) -> (3.0507, -12.1121) centre (3.2628, -11.9) ccw
  line L278 (3.0507, -12.1121) -> (4.3305, -13.392)
  arc A94 (4.3305, -13.392) -> (4.9045, -13.6) centre (4.8416, -12.8778) ccw
  line L279 (4.9045, -13.6) -> (15.0955, -13.6)
  arc A95 (15.0955, -13.6) -> (15.6695, -13.392) centre (15.1584, -12.8778) ccw
  line L280 (15.6695, -13.392) -> (16.9493, -12.1121)
  arc A96 (16.9493, -12.1121) -> (16.7372, -11.6) centre (16.7372, -11.9) ccw
  line L281 (16.7372, -11.6) -> (14.6, -11.6)
  line L282 (14.6, -11.6) -> (14.6, -10.1021)
  line L283 (14.6, -10.1021) -> (17.2021, -7.5)
  line L284 (17.2021, -7.5) -> (22.7979, -7.5)
  line L285 (22.7979, -7.5) -> (25.4, -10.1021)
  line L286 (25.4, -10.1021) -> (25.4, -11.6)
  line L287 (25.4, -11.6) -> (23.2628, -11.6)
  arc A97 (23.2628, -11.6) -> (23.0507, -12.1121) centre (23.2628, -11.9) ccw
  line L288 (23.0507, -12.1121) -> (24.3315, -13.3929)
  arc A98 (24.3315, -13.3929) -> (24.8314, -13.6) centre (24.8314, -12.8929) ccw
  line L289 (24.8314, -13.6) -> (29.5, -13.6)
  arc A99 (29.5, -13.6) -> (30.1, -13) centre (29.5, -13) ccw
  line L290 (30.1, -13) -> (30.1, -8.3314)
  arc A100 (30.1, -8.3314) -> (29.8929, -7.8315) centre (29.3929, -8.3314) ccw
  line L291 (29.8929, -7.8315) -> (28.6121, -6.5507)
  arc A101 (28.6121, -6.5507) -> (28.1, -6.7628) centre (28.4, -6.7628) ccw
  line L292 (28.1, -6.7628) -> (28.1, -8.9)
  line L293 (28.1, -8.9) -> (26.6021, -8.9)
  line L294 (26.6021, -8.9) -> (24, -6.2979)
  line L295 (24, -6.2979) -> (24, -0.7021)
  line L296 (24, -0.7021) -> (26.6021, 1.9)
  line L297 (26.6021, 1.9) -> (28.1, 1.9)
  line L298 (28.1, 1.9) -> (28.1, -0.2372)
  arc A102 (28.1, -0.2372) -> (28.6121, -0.4493) centre (28.4, -0.2372) ccw
  line L299 (28.6121, -0.4493) -> (29.8929, 0.8315)
  arc A103 (29.8929, 0.8315) -> (30.1, 1.3314) centre (29.3929, 1.3314) ccw
  line L300 (30.1, 1.3314) -> (30.1, 6)
  arc A104 (30.1, 6) -> (29.5, 6.6) centre (29.5, 6) ccw
  line L301 (29.5, 6.6) -> (24.9045, 6.6)
  arc A105 (24.9045, 6.6) -> (24.3305, 6.392) centre (24.8416, 5.8778) ccw
  line L302 (24.3305, 6.392) -> (23.0507, 5.1121)
  arc A106 (23.0507, 5.1121) -> (23.2628, 4.6) centre (23.2628, 4.9) ccw
  line L303 (23.2628, 4.6) -> (25.4, 4.6)
  line L304 (25.4, 4.6) -> (25.4, 3.1021)
  line L305 (25.4, 3.1021) -> (22.7979, 0.5)
  line L306 (22.7979, 0.5) -> (17.2021, 0.5)
  line L307 (17.2021, 0.5) -> (14.6, 3.1021)
  line L308 (14.6, 3.1021) -> (14.6, 4.6)
  line L309 (14.6, 4.6) -> (16.7372, 4.6)
  arc A107 (16.7372, 4.6) -> (16.9493, 5.1121) centre (16.7372, 4.9) ccw
  line L310 (16.9493, 5.1121) -> (15.6695, 6.392)
  arc A108 (15.6695, 6.392) -> (15.0955, 6.6) centre (15.1584, 5.8778) ccw
  line L311 (15.0955, 6.6) -> (4.9045, 6.6)
  arc A109 (4.9045, 6.6) -> (4.3305, 6.392) centre (4.8416, 5.8778) ccw
  line L312 (4.3305, 6.392) -> (3.0507, 5.1121)
  arc A110 (3.0507, 5.1121) -> (3.2628, 4.6) centre (3.2628, 4.9) ccw
  line L313 (3.2628, 4.6) -> (5.4, 4.6)
  line L314 (5.4, 4.6) -> (5.4, 3.1021)
  line L315 (5.4, 3.1021) -> (2.7979, 0.5)
  line L316 (2.7979, 0.5) -> (-2.7979, 0.5)
  line L317 (-2.7979, 0.5) -> (-5.4, 3.1021)
  line L318 (-5.4, 3.1021) -> (-5.4, 4.6)
  line L319 (-5.4, 4.6) -> (-3.2628, 4.6)
  arc A111 (-3.2628, 4.6) -> (-3.0507, 5.1121) centre (-3.2628, 4.9) ccw
  line L320 (-3.0507, 5.1121) -> (-4.3305, 6.392)
  arc A112 (-4.3305, 6.392) -> (-4.9045, 6.6) centre (-4.8416, 5.8778) ccw
  line L321 (-4.9045, 6.6) -> (-15.0955, 6.6)
  arc A113 (-15.0955, 6.6) -> (-15.6695, 6.392) centre (-15.1584, 5.8778) ccw
  line L322 (-15.6695, 6.392) -> (-16.9493, 5.1121)
  arc A114 (-16.9493, 5.1121) -> (-16.7372, 4.6) centre (-16.7372, 4.9) ccw
  line L323 (-16.7372, 4.6) -> (-14.6, 4.6)
  line L324 (-14.6, 4.6) -> (-14.6, 3.1021)
  line L325 (-14.6, 3.1021) -> (-17.2021, 0.5)
  line L326 (-17.2021, 0.5) -> (-22.7979, 0.5)
  line L327 (-22.7979, 0.5) -> (-25.4, 3.1021)
  line L328 (-25.4, 3.1021) -> (-25.4, 4.6)
  line L329 (-25.4, 4.6) -> (-23.2628, 4.6)
  arc A115 (-23.2628, 4.6) -> (-23.0507, 5.1121) centre (-23.2628, 4.9) ccw
  line L330 (-23.0507, 5.1121) -> (-24.3305, 6.392)
  arc A116 (-24.3305, 6.392) -> (-24.9045, 6.6) centre (-24.8416, 5.8778) ccw
  line L331 (-24.9045, 6.6) -> (-29.5, 6.6)
  line L332 (16, -6.2979) -> (12.6, -9.6979)
  line L333 (12.6, -9.6979) -> (12.6, -11.6)
  line L334 (12.6, -11.6) -> (7.4, -11.6)
  line L335 (7.4, -11.6) -> (7.4, -9.6979)
  line L336 (7.4, -9.6979) -> (4, -6.2979)
  line L337 (4, -6.2979) -> (4, -0.7021)
  line L338 (4, -0.7021) -> (7.4, 2.6979)
  line L339 (7.4, 2.6979) -> (7.4, 4.6)
  line L340 (7.4, 4.6) -> (12.6, 4.6)
  line L341 (12.6, 4.6) -> (12.6, 2.6979)
  line L342 (12.6, 2.6979) -> (16, -0.7021)
  line L343 (16, -0.7021) -> (16, -6.2979)
  line L344 (-4, -6.2979) -> (-7.4, -9.6979)
  line L345 (-7.4, -9.6979) -> (-7.4, -11.6)
  line L346 (-7.4, -11.6) -> (-12.6, -11.6)
  line L347 (-12.6, -11.6) -> (-12.6, -9.6979)
  line L348 (-12.6, -9.6979) -> (-16, -6.2979)
  line L349 (-16, -6.2979) -> (-16, -0.7021)
  line L350 (-16, -0.7021) -> (-12.6, 2.6979)
  line L351 (-12.6, 2.6979) -> (-12.6, 4.6)
  line L352 (-12.6, 4.6) -> (-7.4, 4.6)
  line L353 (-7.4, 4.6) -> (-7.4, 2.6979)
  line L354 (-7.4, 2.6979) -> (-4, -0.7021)
  line L355 (-4, -0.7021) -> (-4, -6.2979)
  point P0 (-20, -3.5)
  point P1 (20, -3.5)
  point P2 (0, -3.5)
  point P3 (0, -3.5)
  dimension "d47" = 4.2
  dimension "d48" = 4.2
  dimension "d49" = 4.2
  dimension "d50" = 0.1
  dimension "d51" = 0.1
  dimension "d52" = 0.1
  constraint midpoint L20 L30.start
  constraint midpoint L6 L30.end
  constraint coincident P1 A13.centre
  constraint coincident P3 P2
  constraint coincident P0 A19.centre
  constraint tangent A39 L247
  measures "d47" diameter of A13
  measures "d48" diameter of A69
  measures "d49" diameter of A19
extrude "Extrude8" add sketch "Sketch4" against normal blind 2 contours A0 A5 L27 L28 L29 L32 L34 L35 L36 A6 L37 L38 L39 L40 L41 L42 L43 L44 A7 L45 L46 L59 L60 L65 L66 L67 L68 L69 A12 L70 L72 L74 L75 A14 L80 L81 A18 L83 L84 L85 L90 A20 L93 L94 L97 L99 L102 L105 A27 L106 L108 L113 L115 L120 L123 A41 L126 L140 L150 L171 L205 L206 L207 L208 L209 L210 L211 L212 L213 A66 L214 L215 L216 L226 L227 L240 A73 L241 L242 A74 A75 L243 A76 A77 A78 L244 A79 L247 | A0 L34 L59 L74 L85 L140 L205 L213 A66 L214 L216 A73 L241 L243 A76 A77 L244 L247 A113 L322 A114 L323 L324 L325 L326 L327 | A0 L247 A113 L322 A114 L323 L324 L325 L326 L327 L329 A115 L330 A116 | L28 L35 L37 L39 L41 L42 L84 L208 L210 L240 L242 L350 L351 L352 L353 L354 | A0 A16 A26 L107 A36 L125 L151 A54 L163 L247 L329 A115 L330 A116 | L28 L350 L351 L352 L353 L354 | A0 A16 A26 L107 A36 L125 L129 L149 L151 A54 L163 L247 | L28 L60 L65 L80 L83 L97 L99 L106 L113 L115 L123 L338 L339 L340 L341 L342 | L28 L338 L339 L340 L341 L342 | L32 A6 L40 L43 L44 L45 L67 A12 L70 L72 A18 L93 L94 L102 A27 L207 L209 L211 L212 L215 L226 L227 A74 A75 A78 A79 L247 A109 L312 A110 L313 L314 L315 L316 L317 L318 L319 A111 L320 A112 | L247 A109 L312 A110 L313 L314 L315 L316 L317 L318 L319 A111 L320 A112 | A5 A7 L46 L66 L68 L75 A14 L81 L90 A20 L105 L108 L120 A41 L126 L150 L171 L247 L305 L306 L307 L308 L309 A107 L310 A108 | A5 L247 A105 L302 A106 L303 L305 L306 L307 L308 L309 A107 L310 A108 | A5 A21 A28 L112 A31 A34 L116 L138 L175 L247 A105 L302 A106 L303 | A5 A21 A28 L112 A31 A34 L116 L138 L162 L175 L183 L247
extrude "Extrude9" add sketch "Sketch4" along normal blind 3 contours A0 L327 L328 L329 | A0 L247 A113 L322 A114 L323 L324 L325 L326 L327 L329 A115 L330 A116 | L247 A109 L312 A110 L313 L314 L315 L316 L317 L318 L319 A111 L320 A112 | A5 L247 A105 L302 A106 L303 L305 L306 L307 L308 L309 A107 L310 A108 | A5 L303 L304 L305
chamfer "Chamfer1" distance 3 angle 45 3 edges at (20, -0.5, 33) (0, -0.5, 33) (-20, -0.5, 33) measured on face at (20.9326, -3.3305, 33) measured on face at (0.9326, -3.3305, 33) measured on face at (-19.0674, -3.3305, 33)
extrude "Extrude10" add sketch "Sketch4" along normal blind 2 from surface at -60 contours A0 A5 L27 L28 L29 L32 L34 L35 L36 A6 L37 L38 L39 L40 L41 L42 L43 L44 A7 L45 L46 L59 L60 L65 L66 L67 L68 L69 A12 L70 L72 L74 L75 A14 L80 L81 A18 L83 L84 L85 L90 A20 L93 L94 L97 L99 L102 L105 A27 L106 L108 L113 L115 L120 L123 A41 L126 L140 L150 L171 L205 L206 L207 L208 L209 L210 L211 L212 L213 A66 L214 L215 L216 L226 L227 L240 A73 L241 L242 A74 A75 L243 A76 A77 A78 L244 A79 L247 | A0 L34 L59 L74 L85 L140 L205 L213 A66 L214 L216 A73 L241 L243 A76 A77 L244 L247 A113 L322 A114 L323 L324 L325 L326 L327 | A0 L247 A113 L322 A114 L323 L324 L325 L326 L327 L329 A115 L330 A116 | L28 L35 L37 L39 L41 L42 L84 L208 L210 L240 L242 L350 L351 L352 L353 L354 | A0 A16 A26 L107 A36 L125 L151 A54 L163 L247 L329 A115 L330 A116 | L28 L350 L351 L352 L353 L354 | A0 A16 A26 L107 A36 L125 L129 L149 L151 A54 L163 L247 | L28 L60 L65 L80 L83 L97 L99 L106 L113 L115 L123 L338 L339 L340 L341 L342 | L28 L338 L339 L340 L341 L342 | L32 A6 L40 L43 L44 L45 L67 A12 L70 L72 A18 L93 L94 L102 A27 L207 L209 L211 L212 L215 L226 L227 A74 A75 A78 A79 L247 A109 L312 A110 L313 L314 L315 L316 L317 L318 L319 A111 L320 A112 | L247 A109 L312 A110 L313 L314 L315 L316 L317 L318 L319 A111 L320 A112 | A5 A7 L46 L66 L68 L75 A14 L81 L90 A20 L105 L108 L120 A41 L126 L150 L171 L247 L305 L306 L307 L308 L309 A107 L310 A108 | A5 L247 A105 L302 A106 L303 L305 L306 L307 L308 L309 A107 L310 A108 | A5 A21 A28 L112 A31 A34 L116 L138 L175 L247 A105 L302 A106 L303 | A5 A21 A28 L112 A31 A34 L116 L138 L162 L175 L183 L247
extrude "Extrude11" add sketch "Sketch4" against normal blind 3 from surface at -60 contours A0 L327 L328 L329 | A0 L247 A113 L322 A114 L323 L324 L325 L326 L327 L329 A115 L330 A116 | L247 A109 L312 A110 L313 L314 L315 L316 L317 L318 L319 A111 L320 A112 | A5 L247 A105 L302 A106 L303 L305 L306 L307 L308 L309 A107 L310 A108 | A5 L303 L304 L305
extrude "Extrude12" cut sketch "Sketch1" along normal blind 6.6 contours A9
chamfer "Chamfer2" distance 3 angle 45 3 edges at (-20, -0.5, -33) (0, -0.5, -33) (20, -0.5, -33) measured on face at (-19.0674, -3.3305, -33) measured on face at (0.9326, -3.3305, -33) measured on face at (20.9326, -3.3305, -33)
fillet "Fillet5" radius 2 2 edges at (0, -6.5, 28) (0, -6.5, -28)
fillet "Fillet6" radius 5 3 edges at (0, 0, 28) (4, 0, -28) (-23, 0, -28)
fillet "Fillet1" radius 9 1 edges at (-19, 5, -29)
fillet "Fillet7" radius 10.6 1 edges at (-19, 0, -28)
fillet "Fillet8" radius 7 1 edges at (-19, 0, -29)
extrude "Extrude13" cut sketch "Sketch1" along normal blind 7.4 from surface at 6.8 contours A9 | A10
extrude "Extrude14" cut sketch "Sketch1" along normal blind 15 contours L13 A8 | L13 A8 L36 L37 L39
extrude "Extrude15" cut sketch "Sketch1" along normal blind 11 and the other way blind 8 contours L13 A8 A11 | L13 A8 A11 L37 L38 L39 | L13 A8 | A8 L36 L37 L39 | A8 L37 L38 L39
